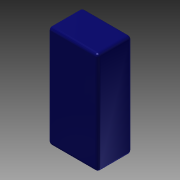
# Autodesk Inventor part: Battery
Saved by Autodesk Inventor 2015 (Build 190159000, 159)
## iProperties
Created: 2016-02-20
Part Number: Battery
Material: Generic
Document SubType Name: Modeling
Designer: 23902
Density: 1 g/cm^3
Appearance: Default
Author: 23902
Autodesk Inventor part; units mm, degrees
ref_plane "YZ Plane" through (0, 0, 0) normal (1, 0, 0) x (0, 1, 0)
ref_plane "XZ Plane" through (0, 0, 0) normal (0, 1, 0) x (-1, 0, 0)
ref_plane "XY Plane" through (0, 0, 0) normal (0, 0, 1) x (1, 0, 0)
sketch "Sketch1" plane through (0, 0, 0) normal (0, 1, 0) x (-1, 0, 0)
  line L0 (17.5, 36) -> (17.5, -36)
  line L1 (17.5, -36) -> (-17.5, -36)
  line L2 (-17.5, -36) -> (-17.5, 36)
  line L3 (-17.5, 36) -> (17.5, 36)
  line L4 (17.5, 36) -> (-17.5, -36) construction
  line L5 (17.5, -36) -> (-17.5, 36) construction
  point P0 (0, 0)
  dimension "d0" = 72
  dimension "d1" = 35
  constraints: 12 end point, 2 midpoint, 2 parallel, 1 perpendicular, 1 vertical
  measures "d0" distance of L0.start L0.end
  measures "d1" distance of L0.end L1.end
extrude "Extrusion1" add sketch "Sketch1" along normal blind 24
fillet "Fillet1" radius 2 12 edges at (0, 24, 36) (-17.5, 12, 36) (-17.5, 24, 0) (-17.5, 0, 0) (17.5, 12, 36) (0, 0, 36) (17.5, 0, 0) (17.5, 24, 0) (17.5, 12, -36) (0, 0, -36) (0, 24, -36) (-17.5, 12, -36)
body "Solid1"
